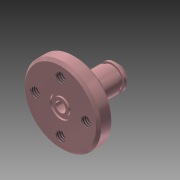
# Autodesk Inventor part: None_Magnet_Extender_Split_Top
Saved by Autodesk Inventor 2015 (Build 190159000, 159)
## iProperties
Created: 2015-01-06
Part Number: None_Magnet_Extender_Split_Top
Material: Aluminum 6061
Document SubType Name: Modeling
Designer: ice
Mass: 1.63117 g
Surface Area: 7.28726 cm^2
Volume: 0.604135 cm^3
Density: 2.7 g/cm^3
Appearance: Aluminum - Flat
Author: ice
Autodesk Inventor part; units mm, degrees
sketch "Sketch1" plane through (0, 0, 0) normal (1, 0, 0) x (0, 1, 0)
  line L0 (20.75, 2.1) -> (20.75, 1.7)
  line L1 (20.4, 1.6) -> (20.4, 0)
  line L2 (31, 0) -> (20.4, 0)
  line L3 (23.4, 7.5) -> (20.4, 7.5)
  line L4 (20.4, 7.5) -> (20.4, 2.2)
  line L5 (20.75, 1.95) -> (20.75, 1.7)
  line L6 (20.75, 1.7) -> (20.75, 1.65)
  line L7 (20.4, 2.2) -> (20.4, 2.15)
  line L8 (20.75, 1.65) -> (20.75, 1.6)
  line L9 (20.75, 1.6) -> (20.4, 1.6)
  line L10 (20.4, 2.15) -> (20.4, 2.1)
  line L11 (20.4, 2.1) -> (20.75, 2.1)
  line L12 (31, 0) -> (32, 0)
  line L13 (32, 0) -> (32, 2.45)
  line L14 (32, 2.45) -> (30.5, 2.45)
  line L15 (30.5, 2.45) -> (30.5, 2.125)
  line L16 (30.5, 2.125) -> (29.7, 2.125)
  line L17 (29.7, 2.125) -> (29.7, 2.45)
  line L18 (29.7, 2.45) -> (26.7, 2.45)
  line L19 (26.7, 2.45) -> (26.7, 2.125)
  line L20 (26.7, 2.125) -> (25.9, 2.125)
  line L21 (25.9, 2.125) -> (25.9, 2.45)
  line L22 (25.9, 2.45) -> (24.4, 2.45)
  line L23 (23.4, 2.5) -> (24.4, 2.5)
  line L24 (24.4, 2.5) -> (24.4, 2.45)
  line L25 (23.4, 2.5) -> (23.4, 7.5)
  line L26 (32, 2.45) -> (31, 2.45)
  line L27 (32, 2.45) -> (32, 1.45)
  point P0 (0, 0)
  dimension "d305" = 3
  dimension "d306" = 5.3
  dimension "d326" = 0.05
  dimension "d329" = 1.6
  dimension "d330" = 0.5
  dimension "d331" = 0.35
  dimension "d344" = 1
  dimension "d345" = 1.5
  dimension "d346" = 0.325
  dimension "d347" = 0.8
  dimension "d348" = 3
  dimension "d349" = 0.325
  dimension "d350" = 0.8
  dimension "d351" = 2.45
  dimension "d353" = 1
  dimension "d354" = 1
  dimension "d355" = 1
  constraints: 56 end point, 10 perpendicular, 5 horizontal, 5 vertical, 4 point on line, 1 collinear
  measures "d305" distance of L3.end L3.start
  measures "d306" distance of L4.end L3.end
  measures "d326" distance of L4.end L7.end
  measures "d329" distance from line of L2 L8.end
  measures "d330" distance of L0.start L8.end
  measures "d331" distance of L8.end L1.start
  measures "d344" distance of L2.start L12.end
  measures "d345" distance of L13.end L14.end
  measures "d346" distance of L14.end L15.end
  measures "d347" distance of L15.end L16.end
  measures "d348" distance of L17.end L18.end
  measures "d349" distance of L18.end L19.end
  measures "d350" distance of L19.end L20.end
  measures "d351" distance between parallel lines of L2 L22
  measures "d353" distance of L23.start L23.end
  measures "d354" distance of L13.end L26.end
  measures "d355" distance of L13.end L27.end
revolve "Revolution1" add sketch "Sketch1" angle 360 about axis through (0, 31, 0) along (0, -1, 0)
sketch "Sketch11" plane through (0, 20.4, 0) normal (0, -1, 0) x (1, 0, 0)
  line L0 (0, 0) -> (0, -5)
  line L1 (0, 0) -> (-5, 0)
  line L2 (0, 0) -> (0, 5)
  line L3 (0, 0) -> (5, 0)
  dimension "d309" = 5
  dimension "d310" = 5
  dimension "d311" = 5
  dimension "d312" = 5
  constraints: 8 end point, 2 horizontal, 2 vertical
  measures "d309" distance of L0.start L0.end
  measures "d310" distance of L0.start L1.end
  measures "d311" distance of L0.start L2.end
  measures "d312" distance of L0.start L3.end
hole "Hole9" at (0, 20.4, -5) at (-5, 20.4, 0) at (0, 20.4, 5) at (5, 20.4, 0) direction (0, 1, 0) diameter 1.9 depth 2 tip angle 118
chamfer "Chamfer6" distance 0.5 angle 45 2 edges at (0, 23.4, -7.5) (0, 20.4, -7.5)
sketch "Sketch12" plane through (0, 20.4, 0) normal (0, -1, 0) x (1, 0, 0)
  circle A0 centre (0, 0) radius 0.9439
  line L0 (0, 0) -> (-21.4854, 21.4854)
  line L1 (0, 0) -> (30.3849, 0) construction
  dimension "d324" = 135
  constraints: 4 end point, 1 centre point, 1 coincident, 1 equal length, 1 horizontal
  measures "d324" angle of L1 L0
ref_plane "Work Plane6" through (0, 20.4, 0) normal (0, -1, 0) x (1, 0, 0)
ref_plane "Work Plane7" through (0, 20.75, 0) normal (0, -1, 0) x (1, 0, 0)
thread "Thread17" size "M2x0.4" class "6H" standard "ANSI Metric M Profile" full length
thread "Thread18" size "M2x0.4" class "6H" standard "ANSI Metric M Profile" full length
thread "Thread19" size "M2x0.4" class "6H" standard "ANSI Metric M Profile" full length
thread "Thread20" size "M2x0.4" class "6H" standard "ANSI Metric M Profile" full length
chamfer "Chamfer8" distance 1 angle 45 1 edges at (0, 32, -2.45)
sketch "Sketch13" plane through (0, 32, 0) normal (0, 1, 0) x (1, 0, 0)
  circle A0 centre (0, 0) radius 1
  dimension "d359" = 2
  constraints: 1 centre point, 1 coincident
  measures "d359" diameter of A0
hole "Hole10" at (0, 32, 0) direction (0, -1, 0) diameter 2 end through all
ref_plane "Work Plane8" through (0, 26.3, 0) normal (0, 1, 0) x (1, 0, 0)
ref_plane "Work Plane9" through (0, 30.1, 0) normal (0, 1, 0) x (1, 0, 0)
body "Solid1"
